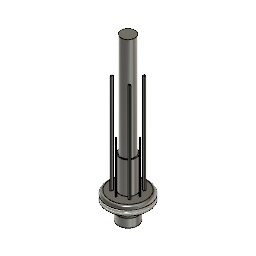
Buoyani-3D-v3 (Autodesk Fusion 360 design; units mm, degrees)
Autodesk Fusion 360 part; units mm, degrees
note: some values were not read from the file. Set by a fixed rule: which face or edge a step refers to.
sketch "Sketch1" plane through (0, 0, 0) normal (0, 0, 1) x (1, 0, 0)
  circle A0 centre (0, 0) radius 25
  dimension "d1" = 50
  constraint coincident A0.centre origin
  measures "d1" diameter of A0
extrude "Extrude1" add sketch "Sketch1" along normal blind 20 makes body 1
extrude "Extrude2" add 1 faces at (-6.7759, -1.242, 20) along direction (0, 0, 1) blind 10 on bodies 1 bodies 1
fillet "Fillet1" radius 4.5 1 faces at (-24.8758, 2.4892, 10) on bodies 1
extrude "Extrude3" add 1 faces at (5.4025, 6.3711, 30) along direction (0, 0, 1) blind 20 on bodies 1 bodies 1
sketch "Sketch2" plane through (0, 0, 50) normal (0, 0, 1) x (-1, 0, 0)
  circle A0 centre (0, 0) radius 20.5
  circle A1 centre (0, 0) radius 45
  dimension "d9" = 90
  constraint coincident A0.centre A1.centre
  measures "d9" diameter of A1
extrude "Extrude4" add sketch "Sketch2" along normal blind 20 separate body makes body 2
extrude "Extrude5" add 1 faces at (5.4025, 6.3711, 50) along direction (0, 0, 1) blind 100 on bodies 1 bodies 1 2
fillet "Fillet2" radius 7.5 1 edges at (41.9547, 16.2727, 70) on bodies 1
sketch "Sketch3" plane through (0, 0, 70) normal (0, 0, 1) x (-1, 0, 0)
  circle A0 centre (0, 0) radius 20.5
  circle A1 centre (0, 0) radius 37.5
  line L0 (-1, -29) -> (1, -29)
  line L1 (1, -29) -> (1, -31)
  line L2 (1, -31) -> (-1, -31)
  line L3 (-1, -31) -> (-1, -29)
  line L4 (-1, -29) -> (1, -31) construction
  line L5 (1, -29) -> (-1, -31) construction
  point P0 (0, -30)
  dimension "d15" = 2
  constraint horizontal L0
  constraint perpendicular L0 L1
  constraint parallel L0 L2
  constraint parallel L1 L3
  constraint coincident L4 P0
  constraint coincident L5 P0
  measures "d15" distance of L1.end L2.end
extrude "Extrude6" add sketch "Sketch3" along normal blind 100 contours L0 L1 L2 L3 bodies 1
move_face "MoveFace1" to x (0.939693, -0.34202, 0) y (0.34202, 0.939693, 0) z (0, 0, 1) at (-10.0558, 1.1527, 0) 1 faces at (0.3333, 29.6667, 170) on bodies 1
move_face "MoveFace2" by (1, -1, 0) 1 faces at (0.3333, 29.6667, 170) on bodies 1
sketch "Sketch4" plane through (0, 0, 70) normal (0, 0, 1) x (-1, 0, 0)
  line L0 (-1, -31) -> (-1, -29)
  line L1 (-1, -29) -> (1, -29)
  line L2 (1, -29) -> (1, -31)
  line L3 (1, -31) -> (-1, -31)
  circle A0 centre (0, 0) radius 20.5
  circle A1 centre (0, 0) radius 37.5
  line L4 (-1, 29) -> (1, 29)
  line L5 (1, 29) -> (1, 31)
  line L6 (1, 31) -> (-1, 31)
  line L7 (-1, 31) -> (-1, 29)
  line L8 (-1, 29) -> (1, 31) construction
  line L9 (1, 29) -> (-1, 31) construction
  point P0 (0, 30)
  dimension "d18" = 2
  constraint horizontal L4
  constraint perpendicular L4 L5
  constraint parallel L4 L6
  constraint parallel L5 L7
  constraint coincident L8 P0
  constraint coincident L9 P0
  measures "d18" distance of L4.end L5.end
extrude "Extrude7" add sketch "Sketch4" along normal blind 10 contours L4 L5 L6 L7 bodies 1
extrude "Extrude8" add 1 faces at (0.3333, -30.3333, 80) along direction (0, 0, 1) blind 90 on bodies 1 bodies 1
sketch "Sketch5" plane through (0, 0, 70) normal (0, 0, 1) x (-1, 0, 0)
  line L0 (-1, 31) -> (1, 31)
  line L1 (1, 31) -> (1, 29)
  line L2 (1, 29) -> (-1, 29)
  line L3 (-1, 29) -> (-1, 31)
  line L4 (-1, -31) -> (-1, -29)
  line L5 (-1, -29) -> (1, -29)
  line L6 (1, -29) -> (1, -31)
  line L7 (1, -31) -> (-1, -31)
  circle A0 centre (0, 0) radius 20.5
  circle A1 centre (0, 0) radius 37.5
  line L8 (29, -1) -> (31, -1)
  line L9 (31, -1) -> (31, 1)
  line L10 (31, 1) -> (29, 1)
  line L11 (29, 1) -> (29, -1)
  line L12 (29, -1) -> (31, 1) construction
  line L13 (31, -1) -> (29, 1) construction
  point P0 (30, 0)
  dimension "d23" = 2
  constraint horizontal L8
  constraint perpendicular L8 L9
  constraint parallel L8 L10
  constraint parallel L9 L11
  constraint coincident L12 P0
  constraint coincident L13 P0
  measures "d23" distance of L9.end L10.end
extrude "Extrude9" add sketch "Sketch5" along normal blind 100 contours L8 L9 L10 L11 bodies 1
sketch "Sketch6" plane through (0, 0, 70) normal (0, 0, 1) x (-1, 0, 0)
  line L0 (29, 1) -> (31, 1)
  line L1 (31, 1) -> (31, -1)
  line L2 (31, -1) -> (29, -1)
  line L3 (29, -1) -> (29, 1)
  line L4 (-1, 31) -> (1, 31)
  line L5 (1, 31) -> (1, 29)
  line L6 (1, 29) -> (-1, 29)
  line L7 (-1, 29) -> (-1, 31)
  line L8 (-1, -31) -> (-1, -29)
  line L9 (-1, -29) -> (1, -29)
  line L10 (1, -29) -> (1, -31)
  line L11 (1, -31) -> (-1, -31)
  circle A0 centre (0, 0) radius 20.5
  circle A1 centre (0, 0) radius 37.5
  line L12 (-31, -1) -> (-29, -1)
  line L13 (-29, -1) -> (-29, 1)
  line L14 (-29, 1) -> (-31, 1)
  line L15 (-31, 1) -> (-31, -1)
  line L16 (-31, -1) -> (-29, 1) construction
  line L17 (-29, -1) -> (-31, 1) construction
  point P0 (-30, 0)
  dimension "d26" = 2
  constraint horizontal L12
  constraint perpendicular L12 L13
  constraint parallel L12 L14
  constraint parallel L13 L15
  constraint coincident L16 P0
  constraint coincident L17 P0
  measures "d26" distance of L13.end L14.end
extrude "Extrude10" add sketch "Sketch6" along normal blind 100 contours L12 L13 L14 L15 bodies 1
box "BoxPrimitive1" add length 4.2328 width 4.5648 height 250 placed x (0, -1, 0) y (1, 0, 0) z (0, 0, 1) at (18.5153, 22.1005, 70) bodies 1
box "BoxPrimitive2" add length 2.8067 width 4.4487 height 250 placed x (0, 1, 0) y (-1, 0, 0) z (0, 0, 1) at (24.4487, -20, 70) bodies 1
move_body "Move1" bodies 1 to x (1, 0, 0) y (0, 1, 0) z (0, 0, 1) at (-30, 30, 0)
box "BoxPrimitive3" add length 6.1207 width 3.3207 height 250 placed x (0, 1, 0) y (-1, 0, 0) z (0, 0, 1) at (-48.3828, 5.5124, 70) bodies 1
box "BoxPrimitive4" add length 3.6957 width 2.7461 height 250 placed x (0, 1, 0) y (-1, 0, 0) z (0, 0, 1) at (-47.2539, 50, 70) bodies 1
move_face "MoveFace3" by (-7.2187, -46.4817, 0) 1 faces at (-30.7379, 20.1532, 150) on bodies 1
cylinder "CylinderPrimitive1" add diameter 35.177 height 260 placed x (1, 0, 0) y (0, 1, 0) z (0, 0, 1) at (-30, 30, 150) bodies 1
thread "Thread1" "ISO Metric profile 105.0 M105x6 6g" major diameter 104.62 minor diameter 97.7258 pitch 6 angle 60 resizes the face on face at (-74.7764, 34.4806, 54.1667) on bodies 1
thread "Thread2" "ISO Metric profile 38.0 M38x1.5 6g" major diameter 37.85 minor diameter 36.1319 pitch 1.5 angle 60 resizes the face on face at (-9.6019, 27.9589, 36.6667) on bodies 1
